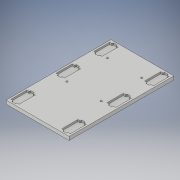
# Autodesk Inventor part: BODY_BOTTOM
Saved by Autodesk Inventor 2017 (Build 210142000, 142)
## iProperties
Created: 2017-08-24
Part Number: BODY_BOTTOM
Material: Generic
Document SubType Name: Modeling
Designer: Alexander Miller
Density: 1 g/cm^3
Appearance: Default
body_A: 150,000 mm
body_B: 90,000 mm
body_C: 5,000 mm
Author: Alexander Miller
Autodesk Inventor part; units mm, degrees
ref_plane "YZ Plane" through (0, 0, 0) normal (1, 0, 0) x (0, 1, 0)
ref_plane "XZ Plane" through (0, 0, 0) normal (0, 1, 0) x (-1, 0, 0)
ref_plane "XY Plane" through (0, 0, 0) normal (0, 0, 1) x (1, 0, 0)
sketch "Sketch4" plane through (0, 0, 0) normal (0, 1, 0) x (-1, 0, 0)
  line L0 (45, 75) -> (-45, 75)
  line L1 (-45, 75) -> (-45, -75)
  line L2 (-45, -75) -> (45, -75)
  line L3 (45, -75) -> (45, 75)
  point P0 (0, 0)
  point P1 (0, -75)
  point P2 (45, 0)
  dimension "d15" = 150
  dimension "d16" = 90
  constraints: 8 end point, 2 midpoint, 2 parallel, 1 horizontal, 1 horizontal alignment, 1 perpendicular, 1 vertical alignment
  measures "d15" distance of L2.end L0.start
  measures "d16" distance of L1.end L2.end
extrude "Extrusion3" add sketch "Sketch4" along normal blind 5
sketch "Sketch5" plane through (0, 5, 0) normal (0, 1, 0) x (1, 0, 0)
  line L0 (-42.5, 70.75) -> (-30.5, 70.75)
  line L1 (-30.5, 70.75) -> (-30.5, 47.75)
  line L2 (-30.5, 47.75) -> (-42.5, 47.75)
  line L3 (-42.5, 47.75) -> (-42.5, 70.75)
  line L4 (-42.5, 17) -> (-30.5, 17)
  line L5 (-30.5, 17) -> (-30.5, -6)
  line L6 (-30.5, -6) -> (-42.5, -6)
  line L7 (-42.5, -6) -> (-42.5, 17)
  line L8 (-42.5, -47.75) -> (-30.5, -47.75)
  line L9 (-30.5, -47.75) -> (-30.5, -70.75)
  line L10 (-30.5, -70.75) -> (-42.5, -70.75)
  line L11 (-42.5, -70.75) -> (-42.5, -47.75)
  line L12 (45, 75) -> (-45, 75) projected
  line L13 (-45, 75) -> (-45, -75) projected
  line L14 (-45, -75) -> (45, -75) projected
  circle A0 centre (-36.5, 0) radius 6 construction
  line L15 (0, 105) -> (0, -105) construction
  line L16 (42.5, 70.75) -> (30.5, 70.75)
  line L17 (30.5, 70.75) -> (30.5, 47.75)
  line L18 (30.5, 47.75) -> (42.5, 47.75)
  line L19 (42.5, 47.75) -> (42.5, 70.75)
  line L20 (42.5, 17) -> (30.5, 17)
  line L21 (30.5, 17) -> (30.5, -6)
  line L22 (30.5, -6) -> (42.5, -6)
  line L23 (42.5, -6) -> (42.5, 17)
  line L24 (42.5, -47.75) -> (30.5, -47.75)
  line L25 (30.5, -47.75) -> (30.5, -70.75)
  line L26 (30.5, -70.75) -> (42.5, -70.75)
  line L27 (42.5, -70.75) -> (42.5, -47.75)
  point P0 (0, 0)
  point P1 (-36.5, 47.75)
  point P2 (-36.5, 17)
  point P3 (-36.5, -6)
  point P4 (-36.5, -47.75)
  dimension "d19" = 23
  dimension "d20" = 12
  dimension "d21" = 4.25
  dimension "d22" = 2.5
  dimension "d23" = 4.25
  constraints: 48 end point, 12 symmetric about line, 6 parallel, 4 equal length, 4 midpoint, 3 horizontal, 3 perpendicular, 3 tangent, 2 vertical alignment, 1 centre point, 1 horizontal alignment
  measures "d19" distance of L2.end L0.start
  measures "d20" distance of L0.start L0.end
  measures "d21" distance between parallel lines of L0 L12
  measures "d22" distance between parallel lines of L3 L13
  measures "d23" distance between parallel lines of L14 L10
extrude "Extrusion4" cut sketch "Sketch5" against normal blind 2.5
sketch "Sketch6" plane through (0, 5, 0) normal (0, 1, 0) x (1, 0, 0)
  line L0 (-39, 72.75) -> (-34, 72.75)
  line L1 (-34, 72.75) -> (-34, 70.75)
  line L2 (-34, 70.75) -> (-39, 70.75)
  line L3 (-39, 70.75) -> (-39, 72.75)
  line L4 (-39, 47.75) -> (-34, 47.75)
  line L5 (-34, 47.75) -> (-34, 45.75)
  line L6 (-34, 45.75) -> (-39, 45.75)
  line L7 (-39, 45.75) -> (-39, 47.75)
  line L8 (-42.5, 70.75) -> (-30.5, 70.75) projected
  line L9 (-30.5, 47.75) -> (-42.5, 47.75) projected
  line L10 (-39, 19) -> (-34, 19)
  line L11 (-34, 19) -> (-34, 17)
  line L12 (-34, 17) -> (-39, 17)
  line L13 (-39, 17) -> (-39, 19)
  line L14 (-39, -6) -> (-34, -6)
  line L15 (-34, -6) -> (-34, -8)
  line L16 (-34, -8) -> (-39, -8)
  line L17 (-39, -8) -> (-39, -6)
  line L18 (-39, -45.75) -> (-34, -45.75)
  line L19 (-34, -45.75) -> (-34, -47.75)
  line L20 (-34, -47.75) -> (-39, -47.75)
  line L21 (-39, -47.75) -> (-39, -45.75)
  line L22 (-39, -70.75) -> (-34, -70.75)
  line L23 (-34, -70.75) -> (-34, -72.75)
  line L24 (-34, -72.75) -> (-39, -72.75)
  line L25 (-39, -72.75) -> (-39, -70.75)
  line L26 (-42.5, 17) -> (-30.5, 17) projected
  line L27 (-30.5, -6) -> (-42.5, -6) projected
  line L28 (-42.5, -47.75) -> (-30.5, -47.75) projected
  line L29 (-30.5, -70.75) -> (-42.5, -70.75) projected
  line L30 (0, 105) -> (0, -105) projected
  line L31 (39, 72.75) -> (34, 72.75)
  line L32 (34, 72.75) -> (34, 70.75)
  line L33 (34, 70.75) -> (39, 70.75)
  line L34 (39, 70.75) -> (39, 72.75)
  line L35 (39, 47.75) -> (34, 47.75)
  line L36 (34, 47.75) -> (34, 45.75)
  line L37 (34, 45.75) -> (39, 45.75)
  line L38 (39, 45.75) -> (39, 47.75)
  line L39 (39, 19) -> (34, 19)
  line L40 (34, 19) -> (34, 17)
  line L41 (34, 17) -> (39, 17)
  line L42 (39, 17) -> (39, 19)
  line L43 (39, -6) -> (34, -6)
  line L44 (34, -6) -> (34, -8)
  line L45 (34, -8) -> (39, -8)
  line L46 (39, -8) -> (39, -6)
  line L47 (39, -45.75) -> (34, -45.75)
  line L48 (34, -45.75) -> (34, -47.75)
  line L49 (34, -47.75) -> (39, -47.75)
  line L50 (39, -47.75) -> (39, -45.75)
  line L51 (39, -70.75) -> (34, -70.75)
  line L52 (34, -70.75) -> (34, -72.75)
  line L53 (34, -72.75) -> (39, -72.75)
  line L54 (39, -72.75) -> (39, -70.75)
  point P0 (0, 0)
  point P1 (-36.5, 70.75)
  point P2 (-36.5, 70.75)
  point P3 (-36.5, 47.75)
  point P4 (-36.5, 47.75)
  point P5 (-36.5, 17)
  point P6 (-36.5, 17)
  point P7 (-36.5, -6)
  point P8 (-36.5, -6)
  point P9 (-36.5, -47.75)
  point P10 (-36.5, -47.75)
  point P11 (-36.5, -70.75)
  point P12 (-36.5, -70.75)
  dimension "d28" = 2
  dimension "d29" = 5
  constraints: 96 end point, 24 symmetric about line, 12 midpoint, 12 parallel, 9 equal length, 6 coincident, 6 collinear, 6 horizontal, 6 perpendicular, 2 point on line
  measures "d28" distance of L2.end L0.start
  measures "d29" distance of L0.start L0.end
extrude "Extrusion5" cut sketch "Sketch6" against normal up to surface (2.5 mm away)
fillet "Fillet1" radius 0.75 24 edges at (-39, 3.75, -70.75) (-34, 3.75, -70.75) (-39, 3.75, -47.75) (-34, 3.75, -47.75) (-39, 3.75, -17) (-34, 3.75, -17) (-39, 3.75, 6) (-34, 3.75, 6) (-39, 3.75, 47.75) (-34, 3.75, 47.75) (-39, 3.75, 70.75) (-34, 3.75, 70.75) (34, 3.75, -70.75) (39, 3.75, -70.75) (34, 3.75, -47.75) (39, 3.75, -47.75) (34, 3.75, -17) (39, 3.75, -17) (34, 3.75, 6) (39, 3.75, 6) (34, 3.75, 47.75) (39, 3.75, 47.75) (34, 3.75, 70.75) (39, 3.75, 70.75)
sketch "Sketch7" plane through (0, 5, 0) normal (0, 1, 0) x (1, 0, 0)
  line L0 (-28, 73) -> (28, 73) construction
  line L1 (28, 73) -> (28, -12) construction
  line L2 (28, -12) -> (-28, -12) construction
  line L3 (-28, -12) -> (-28, 73) construction
  line L4 (45, 75) -> (-45, 75) projected
  circle A0 centre (-24.5, 49.5) radius 1.25
  circle A1 centre (-24.5, -8.5) radius 1.25
  circle A2 centre (24.5, 49.5) radius 1.25
  circle A3 centre (24.5, -8.5) radius 1.25
  point P0 (0, 0)
  point P1 (0, -12)
  dimension "d33" = 85
  dimension "d34" = 56
  dimension "d35" = 2
  dimension "d36" = 2.5
  dimension "d37" = 3.5
  dimension "d38" = 3.5
  dimension "d39" = 3.5
  dimension "d40" = 58
  constraints: 8 end point, 4 centre point, 3 equal radius, 3 vertical alignment, 2 horizontal alignment, 2 parallel, 1 horizontal, 1 midpoint, 1 perpendicular
  measures "d33" distance of L2.end L0.start
  measures "d34" distance of L0.start L0.end
  measures "d35" distance between parallel lines of L4 L0
  measures "d36" diameter of A0
  measures "d37" distance from line of L2 A3.centre
  measures "d38" distance from line of L1 A3.centre
  measures "d39" distance from line of L3 A1.centre
  measures "d40" distance of A0.centre A1.centre
extrude "Extrusion6" cut sketch "Sketch7" against normal through all
sketch "Sketch8" plane through (0, 0, 0) normal (0, -1, 0) x (1, 0, 0)
  circle A0 centre (24.5, -49.5) radius 2.1
  circle A1 centre (-24.5, -49.5) radius 2.1
  circle A2 centre (-24.5, 8.5) radius 2.1
  circle A3 centre (24.5, 8.5) radius 2.1
  circle A4 centre (24.5, -49.5) radius 1.25 projected
  circle A5 centre (-24.5, -49.5) radius 1.25 projected
  circle A6 centre (-24.5, 8.5) radius 1.25 projected
  circle A7 centre (24.5, 8.5) radius 1.25 projected
  point P0 (0, 0)
  dimension "d43" = 4.2
  constraints: 4 centre point, 4 concentric, 3 equal radius
  measures "d43" diameter of A0
extrude "Extrusion7" cut sketch "Sketch8" against normal blind 2
equation "\"d15\" = body_A"
equation "\"d16\" = body_B"
equation "\"d17\" = body_C"
equation "\"d19\" = servo_A"
equation "\"d20\" = servo_B"
equation "\"d21\" = -0.5 * servo_A + 0.5 * servo_D"
equation "\"d22\" = 0.5 * body_C"
equation "\"d23\" = d21"
equation "\"d26\" = 0.5 * body_C"
equation "\"body_A\" = 150"
equation "\"body_B\" = 90"
equation "\"body_C\" = 5"
equation "\"body_D\" = 0.25 * servo_D"
equation "\"body_E\" = 0.25 * servo_D"
equation "\"servo_A\" = 23"
equation "\"servo_B\" = 12"
equation "\"servo_D\" = 31.5"
body "Solid2"
